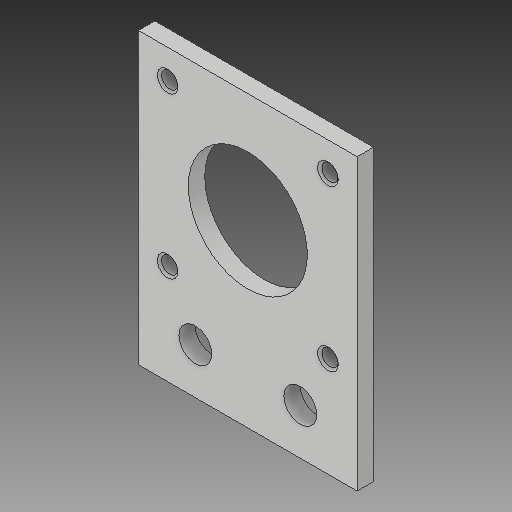
# Autodesk Inventor part: MOTOR MOUNT
Saved by Autodesk Inventor 2018 (Build 220112000, 112)
## iProperties
Created: 2018-10-14
Part Number: MOTOR MOUNT
Material: Generic
Document SubType Name: Modeling
Designer: Matthew Morey
Density: 1 g/cm^3
Appearance: Default
Author: Matthew Morey
Autodesk Inventor part; units mm, degrees
ref_plane "YZ Plane" through (0, 0, 0) normal (1, 0, 0) x (0, 1, 0)
ref_plane "XZ Plane" through (0, 0, 0) normal (0, 1, 0) x (-1, 0, 0)
ref_plane "XY Plane" through (0, 0, 0) normal (0, 0, 1) x (1, 0, 0)
sketch "Sketch1" plane through (0, 0, 0) normal (0, 0, 1) x (1, 0, 0)
  line L0 (-21.15, 28) -> (21.15, 28)
  line L1 (21.15, 28) -> (21.15, -28)
  line L2 (21.15, -28) -> (-21.15, -28)
  line L3 (-21.15, -28) -> (-21.15, 28)
  point P0 (0, 0)
  dimension "d0" = 56
  dimension "d1" = 42.3
  dimension "d2" = 21.15
  dimension "d3" = 28
  dimension "d44" = 21.15
  constraints: 8 end point, 2 parallel, 1 horizontal, 1 perpendicular
  measures "d0" distance between parallel lines of L2 L0
  measures "d1" distance of L0.start L0.end
  measures "d2" distance from line of point (0, 0) L1
  measures "d3" distance from line of point (0, 0) L2
  measures "d44" distance from line of point (0, 0) L3
extrude "Extrusion1" add sketch "Sketch1" along normal blind 3.175
sketch "Sketch2" plane through (0, 0, 3.175) normal (0, 0, 1) x (1, 0, 0)
  circle A0 centre (-15.499, 22.359) radius 1.5875
  circle A1 centre (15.499, 22.359) radius 1.5875
  line L0 (21.15, 28) -> (-21.15, 28) projected
  line L1 (-21.15, 28) -> (-21.15, -28) projected
  line L2 (21.15, -28) -> (21.15, 28) projected
  circle A2 centre (-15.509, -8.635) radius 1.5875
  circle A3 centre (15.509, -8.635) radius 1.5875
  point P0 (0, 0)
  dimension "d6" = 3.175
  dimension "d7" = 5.641
  dimension "d8" = 5.641
  dimension "d9" = 5.651
  dimension "d10" = 5.651
  dimension "d11" = 3.175
  dimension "d45" = 3.175
  dimension "d46" = 3.175
  dimension "d47" = 5.641
  dimension "d48" = 5.641
  dimension "d49" = 36.635
  dimension "d50" = 36.635
  constraints: 4 centre point
  measures "d6" diameter of A0
  measures "d7" distance from line of L0 A0.centre
  measures "d8" distance from line of L0 A1.centre
  measures "d9" distance from line of L1 A0.centre
  measures "d10" distance from line of L2 A1.centre
  measures "d11" diameter of A1
  measures "d45" diameter of A2
  measures "d46" diameter of A3
  measures "d47" distance from line of L1 A2.centre
  measures "d48" distance from line of L2 A3.centre
  measures "d49" distance from line of L0 A2.centre
  measures "d50" distance from line of L0 A3.centre
hole "Hole1" at (-15.499, 22.359, 3.175) at (15.499, 22.359, 3.175) at (-15.509, -8.635, 3.175) at (15.509, -8.635, 3.175) direction (0, 0, -1) diameter 3.175 end through all countersink diameter 4 countersink angle 90
sketch "Sketch3" plane through (0, 0, 3.175) normal (0, 0, 1) x (1, 0, 0)
  circle A0 centre (-10.15, -19.15) radius 3.175
  circle A1 centre (10.15, -19.15) radius 3.175
  line L0 (-21.15, -28) -> (21.15, -28) projected
  line L1 (21.15, -28) -> (21.15, 28) projected
  line L2 (-21.15, 28) -> (-21.15, -28) projected
  line L3 (21.15, 28) -> (-21.15, 28) projected
  point P0 (0, 0)
  dimension "d19" = 6.35
  dimension "d20" = 6.35
  dimension "d22" = 11
  dimension "d23" = 11
  dimension "d25" = 47.15
  dimension "d26" = 47.15
  constraints: 2 centre point
  measures "d19" diameter of A0
  measures "d20" diameter of A1
  measures "d22" distance from line of A1.centre L1
  measures "d23" distance from line of L2 A0.centre
  measures "d25" distance from line of L3 A0.centre
  measures "d26" distance from line of L3 A1.centre
hole "Hole2" at (-10.15, -19.15, 3.175) at (10.15, -19.15, 3.175) direction (0, 0, -1) diameter 6.35 end through all
sketch "Sketch5" plane through (0, 0, 0) normal (0, 0, -1) x (-1, 0, 0)
  circle A0 centre (0, 6.756) radius 11.5
  line L0 (21.15, 28) -> (-21.15, 28) projected
  line L1 (21.15, -28) -> (21.15, 28) projected
  point P0 (0, 0)
  dimension "d39" = 23
  dimension "d40" = 21.244
  dimension "d41" = 21.15
  constraints: 1 centre point
  measures "d39" diameter of A0
  measures "d40" distance from line of A0.centre L0
  measures "d41" distance from line of L1 A0.centre
extrude "Extrusion3" cut sketch "Sketch5" against normal through all
body "Solid1"
